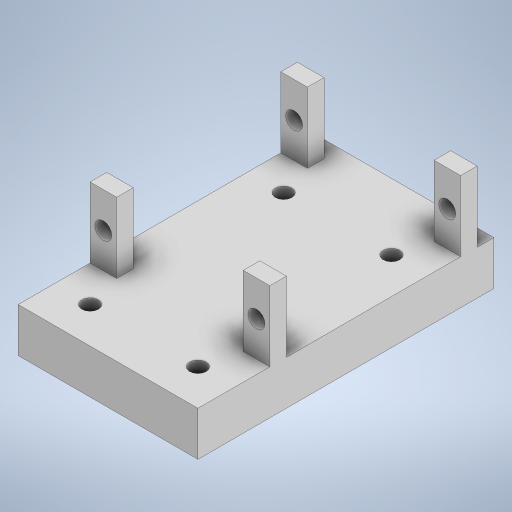
# Autodesk Inventor part: Base_to_servo_mount
Saved by Autodesk Inventor 2023 (Build 270158000, 158)
## iProperties
Created: 2023-02-21
Part Number: Base_to_servo_mount
Material: Ogólny
Document SubType Name: Modeling
Designer: kamil
Density: 1 g/cm^3
Appearance: Domyślna
Author: kamil
Autodesk Inventor part; units mm, degrees
ref_plane "YZ Plane" through (0, 0, 0) normal (1, 0, 0) x (0, 1, 0)
ref_plane "XZ Plane" through (0, 0, 0) normal (0, 1, 0) x (-1, 0, 0)
ref_plane "XY Plane" through (0, 0, 0) normal (0, 0, 1) x (1, 0, 0)
sketch "Szkic1" plane through (0, 0, 0) normal (0, 1, 0) x (-1, 0, 0)
  line L0 (16.25, 26.75) -> (-16.25, 26.75)
  line L1 (-16.25, 26.75) -> (-16.25, -26.75)
  line L2 (-16.25, -26.75) -> (16.25, -26.75)
  line L3 (16.25, -26.75) -> (16.25, 26.75)
  point P0 (0, 0)
  point P1 (0, 0)
  point P2 (0, 26.75)
  dimension "d0" = 32.5
  dimension "d1" = 53.5
  dimension "d2" = 26.75
  dimension "d3" = 16.25
  constraints: 8 end point, 2 parallel, 1 coincident, 1 horizontal, 1 midpoint, 1 perpendicular
  measures "d0" distance of L2.end L1.end
  measures "d1" distance of L1.end L0.end
  measures "d2" distance of point (0, 0) point (0, 26.75)
  measures "d3" distance from line of L3 point (0, 0)
extrude "Wyciągnięcie proste1" add sketch "Szkic1" along normal blind 8
sketch "Szkic2" plane through (0, 8, 0) normal (0, 1, 0) x (1, 0, 0)
  line L0 (-16.25, -26.75) -> (16.25, -26.75) projected
  line L1 (-16.25, 26.75) -> (-16.25, -26.75) projected
  line L2 (16.25, -26.75) -> (16.25, 26.75) projected
  line L3 (-16.25, -13.75) -> (-11.45, -13.75)
  line L4 (-11.45, -13.75) -> (-11.45, -10.75)
  line L5 (-11.45, -10.75) -> (-16.25, -10.75)
  line L6 (-16.25, -10.75) -> (-16.25, -13.75)
  line L7 (16.25, -13.75) -> (11.45, -13.75)
  line L8 (11.45, -13.75) -> (11.45, -10.75)
  line L9 (11.45, -10.75) -> (16.25, -10.75)
  line L10 (16.25, -10.75) -> (16.25, -13.75)
  line L11 (-16.25, 23.75) -> (-11.45, 23.75)
  line L12 (-11.45, 23.75) -> (-11.45, 20.75)
  line L13 (-11.45, 20.75) -> (-16.25, 20.75)
  line L14 (-16.25, 20.75) -> (-16.25, 23.75)
  line L15 (16.25, 20.75) -> (11.45, 20.75)
  line L16 (11.45, 20.75) -> (11.45, 23.75)
  line L17 (11.45, 23.75) -> (16.25, 23.75)
  line L18 (16.25, 23.75) -> (16.25, 20.75)
  point P0 (0, 0)
  dimension "d7" = 4.8
  dimension "d8" = 3
  dimension "d9" = 4.8
  dimension "d10" = 3
  dimension "d11" = 4.8
  dimension "d12" = 3
  dimension "d13" = 4.8
  dimension "d14" = 3
  dimension "d15" = 13
  dimension "d16" = 13
  dimension "d17" = 3
  dimension "d18" = 3
  constraints: 32 end point, 8 parallel, 4 horizontal, 4 perpendicular, 4 point on line
  measures "d7" distance of L5.end L4.end
  measures "d8" distance of L4.end L3.end
  measures "d9" distance of L8.end L9.end
  measures "d10" distance of L7.end L8.end
  measures "d11" distance of L12.end L13.end
  measures "d12" distance of L11.end L12.end
  measures "d13" distance of L16.end L17.end
  measures "d14" distance of L15.end L16.end
  measures "d15" distance of L0.start L3.start
  measures "d16" distance of L0.end L7.start
  measures "d17" distance of L1.start L11.start
  measures "d18" distance of L2.end L17.end
extrude "Wyciągnięcie proste2" add sketch "Szkic2" along normal blind 12.7
sketch "Szkic3" plane through (-16.25, 8, 13.75) normal (0, 0, 1) x (1, 0, 0)
  circle A0 centre (2.4, 6.3) radius 1.525
  circle A1 centre (30.1, 6.3) radius 1.525
  line L0 (0, 0) -> (32.5, 0) projected
  line L1 (4.8, 0) -> (4.8, 12.7) projected
  line L2 (32.5, 0) -> (32.5, 12.7) projected
  point P0 (16.25, -8)
  dimension "d21" = 3.05
  dimension "d22" = 3.05
  dimension "d23" = 6.3
  dimension "d24" = 6.3
  dimension "d25" = 2.4
  dimension "d26" = 2.4
  constraints: 2 centre point
  measures "d21" diameter of A0
  measures "d22" diameter of A1
  measures "d23" distance from line of A0.centre L0
  measures "d24" distance from line of L0 A1.centre
  measures "d25" distance from line of L1 A0.centre
  measures "d26" distance from line of L2 A1.centre
sketch "Szkic4" plane through (-16.25, 8, -20.75) normal (0, 0, 1) x (1, 0, 0)
  point P0 (16.25, -8)
sketch "Szkic5" plane through (-11.45, 8, -23.75) normal (0, 0, -1) x (-1, 0, 0)
  circle A0 centre (-25.3, 6.3) radius 1.525
  circle A1 centre (2.4, 6.3) radius 1.525
  line L0 (-27.7, 0) -> (4.8, 0) projected
  line L1 (-22.9, 0) -> (-22.9, 12.7) projected
  line L2 (4.8, 0) -> (4.8, 12.7) projected
  point P0 (-11.45, -8)
  dimension "d27" = 3.05
  dimension "d28" = 3.05
  dimension "d29" = 6.3
  dimension "d30" = 2.4
  dimension "d31" = 2.4
  dimension "d32" = 6.3
  constraints: 2 centre point
  measures "d27" diameter of A0
  measures "d28" diameter of A1
  measures "d29" distance from line of L0 A0.centre
  measures "d30" distance from line of L1 A0.centre
  measures "d31" distance from line of L2 A1.centre
  measures "d32" distance from line of L0 A1.centre
extrude "Wyciągnięcie proste3" cut sketch "Szkic3" against normal blind 3
extrude "Wyciągnięcie proste4" cut sketch "Szkic5" against normal blind 3
sketch "Szkic6" plane through (0, 8, 0) normal (0, 1, 0) x (1, 0, 0)
  circle A0 centre (-9.75, 14.75) radius 1.5
  line L0 (16.25, 26.75) -> (-16.25, 26.75) projected
  line L1 (-16.25, 20.75) -> (-16.25, -10.75) projected
  circle A1 centre (-9.75, -20.25) radius 1.5
  line L2 (0, 26.75) -> (0, -26.75)
  line L3 (-16.25, -26.75) -> (16.25, -26.75) projected
  circle A2 centre (9.75, 14.75) radius 1.5
  circle A3 centre (9.75, -20.25) radius 1.5
  point P0 (0, 0)
  dimension "d37" = 3
  dimension "d38" = 12
  dimension "d39" = 6.5
  dimension "d42" = 35
  dimension "d49" = 9.75
  constraints: 4 centre point, 2 end point, 2 midpoint, 2 symmetric about line, 1 vertical, 4 other
  measures "d37" diameter of A0
  measures "d38" distance from line of L0 A0.centre
  measures "d39" distance from line of L1 A0.centre
  measures "d42" distance of A0.centre A1.centre
  measures "d49" distance from line of A0.centre L2
extrude "Wyciągnięcie proste5" cut sketch "Szkic6" against normal blind 10
